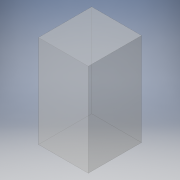
# Autodesk Inventor part: maxVolume
Saved by Autodesk Inventor 2016 SP1 (Build 200210100, 210)
## iProperties
Created: 2016-01-12
Part Number: maxVolume
Material: Polycarbonate, Clear
Document SubType Name: Modeling
Designer: steele
Density: 1.2 g/cm^3
Appearance: Polycarbonate - Clear
Author: steele
Autodesk Inventor part; units mm, degrees
ref_plane "YZ Plane" through (0, 0, 0) normal (1, 0, 0) x (0, 1, 0)
ref_plane "XZ Plane" through (0, 0, 0) normal (0, 1, 0) x (-1, 0, 0)
ref_plane "XY Plane" through (0, 0, 0) normal (0, 0, 1) x (1, 0, 0)
sketch "Sketch2" plane through (0, 0, 0) normal (0, 1, 0) x (-1, 0, 0)
  line L0 (368.3, 393.7) -> (-368.3, 393.7)
  line L1 (-368.3, 393.7) -> (-368.3, -393.7)
  line L2 (-368.3, -393.7) -> (368.3, -393.7)
  line L3 (368.3, -393.7) -> (368.3, 393.7)
  line L4 (368.3, 393.7) -> (-368.3, -393.7) construction
  line L5 (-368.3, 393.7) -> (368.3, -393.7) construction
  point P0 (0, 0)
  dimension "d4" = 736.6
  dimension "d5" = 787.4
  constraints: 12 end point, 2 midpoint, 2 parallel, 1 horizontal, 1 perpendicular
  measures "d4" distance of L0.start L0.end
  measures "d5" distance of L2.end L0.start
extrude "Extrusion1" add sketch "Sketch2" along normal blind 1371.6
equation "\"d4\" = width"
equation "\"d5\" = length"
equation "\"d6\" = height"
equation "\"width\" = -length + 0.5 * perimeter"
equation "\"length\" = 787.4"
equation "\"height\" = 1371.6"
equation "\"perimeter\" = 3048"
body "Solid1"
